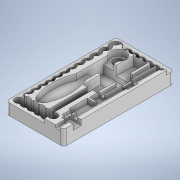
# Autodesk Inventor part: tool box
Saved by Autodesk Inventor 2020 (Build 240168000, 168)
## iProperties
Created: 2020-01-06
Part Number: tool box
Material: Générique
Document SubType Name: Modeling
Designer: damien
Density: 1 g/cm^3
Appearance: Par défaut
Author: damien
Autodesk Inventor part; units mm, degrees
ref_plane "YZ Plane" through (0, 0, 0) normal (1, 0, 0) x (0, 1, 0)
ref_plane "XZ Plane" through (0, 0, 0) normal (0, 1, 0) x (-1, 0, 0)
ref_plane "XY Plane" through (0, 0, 0) normal (0, 0, 1) x (1, 0, 0)
sketch "Esquisse1" plane through (0, 0, 0) normal (0, 1, 0) x (-1, 0, 0)
  line L0 (-50, -95.5) -> (50, -95.5)
  line L1 (50, -95.5) -> (50, 95.5)
  line L2 (50, 95.5) -> (-50, 95.5)
  line L3 (-50, 95.5) -> (-50, -95.5)
  line L4 (-50, -95.5) -> (50, 95.5) construction
  line L5 (50, -95.5) -> (-50, 95.5) construction
  point P0 (0, 0)
  dimension "d0" = 100
  dimension "d1" = 191
  constraints: 12 end point, 2 midpoint, 2 parallel, 1 horizontal, 1 perpendicular
  measures "d0" distance of L0.start L0.end
  measures "d1" distance of L0.end L1.end
extrude "Extrusion1" add sketch "Esquisse1" along normal blind 26.5
fillet "Congé1" radius 5 4 edges at (50, 13.25, 95.5) (50, 13.25, -95.5) (-50, 13.25, -95.5) (-50, 13.25, 95.5)
sketch "Esquisse2" plane through (0, 26.5, 0) normal (0, 1, 0) x (1, 0, 0)
  line L0 (-50, -95.5) -> (16.5, -95.5)
  line L1 (50, 95.5) -> (-50, 95.5)
  line L2 (-50, 95.5) -> (-50, -95.5)
  line L3 (50, 95.5) -> (-50, 95.5) projected
  line L4 (-50, 95.5) -> (-50, -95.5) projected
  line L5 (-50, -95.5) -> (50, -95.5) projected
  line L6 (-37, -80) -> (16.5, -80)
  line L7 (50, 82.5) -> (-37, 82.5)
  line L8 (-37, 82.5) -> (-37, -80)
  line L9 (16.5, -95.5) -> (16.5, -80)
  line L10 (50, 82.5) -> (50, 95.5)
  line L11 (50, -95.5) -> (50, 95.5) projected
  point P0 (0, 0)
  point P1 (45, 95.5)
  point P2 (-45, 95.5)
  point P3 (-50, 90.5)
  point P4 (45, -95.5)
  point P5 (50, -90.5)
  point P6 (50, 90.5)
  dimension "d5" = 15.5
  dimension "d7" = 13
  dimension "d8" = 13
  dimension "d9" = 66.5
  constraints: 19 end point, 4 parallel, 2 horizontal, 2 perpendicular, 1 collinear
  measures "d5" distance between parallel lines of L0 L6
  measures "d7" distance between parallel lines of L2 L8
  measures "d8" distance from line of point (45, 95.5) L7
  measures "d9" distance of L0.start L0.end
extrude "Extrusion2" cut sketch "Esquisse2" against normal blind 7 contours L2 L1 L10 L7 L8 L6 L9 L0
sketch "Esquisse4" plane through (0, 26.5, 0) normal (0, 1, 0) x (1, 0, 0)
  arc A0 (14, -87.1056) -> (14, -79.8944) centre (20, -83.5) ccw
  line L0 (50, -95.5) -> (50, 82.5) projected
  line L1 (16.5, -95.5) -> (50, -95.5) projected
  arc A1 (-34, -79.8944) -> (-34, -87.1056) centre (-40, -83.5) ccw
  line L2 (8, -83.5) -> (-4, -83.5) construction
  line L3 (-4, -83.5) -> (-16, -83.5) construction
  line L4 (-16, -83.5) -> (-28, -83.5) construction
  line L5 (-28, -83.5) -> (-40, -83.5) construction
  line L6 (-50, -90.5) -> (-50, 90.5) projected
  arc A2 (-34, -87.1056) -> (-22, -87.1056) centre (-28, -83.5) ccw
  arc A3 (-22, -79.8944) -> (-34, -79.8944) centre (-28, -83.5) ccw
  arc A4 (-22, -87.1056) -> (-10, -87.1056) centre (-16, -83.5) ccw
  arc A5 (-10, -79.8944) -> (-22, -79.8944) centre (-16, -83.5) ccw
  arc A6 (-10, -87.1056) -> (2, -87.1056) centre (-4, -83.5) ccw
  arc A7 (2, -79.8944) -> (-10, -79.8944) centre (-4, -83.5) ccw
  arc A8 (2, -87.1056) -> (14, -87.1056) centre (8, -83.5) ccw
  arc A9 (14, -79.8944) -> (2, -79.8944) centre (8, -83.5) ccw
  point P0 (0, 0)
  point P1 (50, -90.5)
  point P2 (45, -95.5)
  point P3 (-50, -95.5)
  point P4 (-50, 95.5)
  dimension "d12" = 30
  dimension "d13" = 14
  dimension "d14" = 12
  dimension "d16" = 12
  dimension "d17" = 12
  dimension "d18" = 12
  dimension "d19" = 12
  dimension "d20" = 12
  dimension "d21" = 10
  dimension "d25" = 14
  dimension "d26" = 7
  dimension "d27" = 7
  dimension "d28" = 7
  dimension "d29" = 7
  dimension "d30" = 7
  dimension "d31" = 7
  dimension "d32" = 7
  dimension "d33" = 7
  constraints: 20 point on circle, 10 centre point, 8 end point, 4 horizontal alignment, 3 collinear, 1 horizontal
  measures "d12" distance from line of L0 A0.centre
  measures "d13" diameter of A0
  measures "d14" distance from line of L1 A0.centre
  measures "d16" distance of A0.centre L2.start
  measures "d17" distance of L2.end L2.start
  measures "d18" distance of L2.end L3.end
  measures "d19" distance of L3.end L4.end
  measures "d20" distance of L4.end L5.end
  measures "d21" distance from line of L6 L5.end
  measures "d25" diameter of A1
  measures "d26" radius of A3
  measures "d27" radius of A2
  measures "d28" radius of A4
  measures "d29" radius of A5
  measures "d30" radius of A6
  measures "d31" radius of A7
  measures "d32" radius of A8
  measures "d33" radius of A9
extrude "Extrusion3" cut sketch "Esquisse4" against normal blind 26
fillet "Congé2" radius 2 10 edges at (-34, 13.5, 79.8944) (-22, 13.5, 79.8944) (-10, 13.5, 79.8944) (2, 13.5, 79.8944) (14, 13.5, 79.8944) (14, 10, 87.1056) (2, 10, 87.1056) (-10, 10, 87.1056) (-22, 10, 87.1056) (-34, 10, 87.1056)
fillet "Congé3" [suppressed]
sketch "Esquisse5" plane through (0, 26.5, 0) normal (0, 1, 0) x (1, 0, 0)
  arc A0 (-40.2854, -61.75) -> (-36.7146, -61.75) centre (-38.5, -68) ccw
  arc A1 (-36.619, 74.0454) -> (-40.381, 74.0454) centre (-38.5, 83) ccw
  arc A2 (-37, -77.1754) -> (-34, -87.1056) centre (-40, -83.5) ccw projected
  line L0 (-50, -90.5) -> (-50, 90.5) projected
  arc A3 (-36.7146, -61.75) -> (-36.7146, -49.25) centre (-38.5, -55.5) ccw
  arc A4 (-40.2854, -49.25) -> (-40.2854, -61.75) centre (-38.5, -55.5) ccw
  arc A5 (-36.7146, -49.25) -> (-36.7146, -36.75) centre (-38.5, -43) ccw
  arc A6 (-40.2854, -36.75) -> (-40.2854, -49.25) centre (-38.5, -43) ccw
  arc A7 (-36.7146, -36.75) -> (-36.7146, -24.25) centre (-38.5, -30.5) ccw
  arc A8 (-40.2854, -24.25) -> (-40.2854, -36.75) centre (-38.5, -30.5) ccw
  arc A9 (-36.7146, -24.25) -> (-36.7146, -11.75) centre (-38.5, -18) ccw
  arc A10 (-40.2854, -11.75) -> (-40.2854, -24.25) centre (-38.5, -18) ccw
  arc A11 (-36.7146, -11.75) -> (-36.7146, 0.75) centre (-38.5, -5.5) ccw
  arc A12 (-40.2854, 0.75) -> (-40.2854, -11.75) centre (-38.5, -5.5) ccw
  arc A13 (-36.7146, 0.75) -> (-36.9688, 13.3171) centre (-38.5, 7) ccw
  arc A14 (-40.0312, 13.3171) -> (-40.2854, 0.75) centre (-38.5, 7) ccw
  arc A15 (-36.9688, 13.3171) -> (-36.613, 27.0946) centre (-38.5, 20.25) ccw
  arc A16 (-40.387, 27.0946) -> (-40.0312, 13.3171) centre (-38.5, 20.25) ccw
  arc A17 (-36.613, 27.0946) -> (-36.5496, 41.3883) centre (-38.5, 34.25) ccw
  arc A18 (-40.4504, 41.3883) -> (-40.387, 27.0946) centre (-38.5, 34.25) ccw
  arc A19 (-36.5496, 41.3883) -> (-36.2736, 57.038) centre (-38.5, 49.25) ccw
  arc A20 (-40.7264, 57.038) -> (-40.4504, 41.3883) centre (-38.5, 49.25) ccw
  arc A21 (-36.2736, 57.038) -> (-36.619, 74.0454) centre (-38.5, 65.5) ccw
  arc A22 (-40.381, 74.0454) -> (-40.7264, 57.038) centre (-38.5, 65.5) ccw
  point P0 (0, 0)
  point P1 (-35.3333, -88.7175)
  point P2 (-35.3333, -78.2825)
  point P3 (-50, -95.5)
  point P4 (-50, 95.5)
  dimension "d38" = 13
  dimension "d39" = 15.5
  dimension "d40" = 7
  dimension "d41" = 11.5
  dimension "d42" = 12.5
  dimension "d43" = 12.5
  dimension "d44" = 12.5
  dimension "d45" = 12.5
  dimension "d46" = 12.5
  dimension "d47" = 6.5
  dimension "d49" = 12.5
  dimension "d51" = 13.25
  dimension "d52" = 14
  dimension "d55" = 15
  dimension "d57" = 16.25
  dimension "d58" = 18.3
  dimension "d59" = 17.5
  dimension "d60" = 6.5
  dimension "d61" = 6.5
  dimension "d62" = 7.1
  dimension "d63" = 7.4
  dimension "d64" = 8.1
  dimension "d65" = 8.75
  constraints: 44 point on circle, 22 centre point, 13 equal radius, 11 vertical alignment
  measures "d38" diameter of A0
  measures "d39" vertical distance of A2.centre A0.centre
  measures "d40" radius of A2
  measures "d41" distance from line of L0 A0.centre
  measures "d42" distance of A3.centre A0.centre
  measures "d43" distance of A5.centre A3.centre
  measures "d44" distance of A7.centre A5.centre
  measures "d45" distance of A9.centre A7.centre
  measures "d46" distance of A11.centre A9.centre
  measures "d47" radius of A3
  measures "d49" distance of A13.centre A11.centre
  measures "d51" distance of A13.centre A15.centre
  measures "d52" distance of A15.centre A17.centre
  measures "d55" distance of A17.centre A19.centre
  measures "d57" distance of A19.centre A21.centre
  measures "d58" diameter of A1
  measures "d59" distance of A21.centre A1.centre
  measures "d60" radius of A12
  measures "d61" radius of A14
  measures "d62" radius of A16
  measures "d63" radius of A18
  measures "d64" radius of A20
  measures "d65" radius of A22
extrude "Extrusion4" cut sketch "Esquisse5" against normal blind 26
fillet "Congé4" radius 2 10 edges at (-36.7146, 13.5, 49.25) (-36.7146, 13.5, 36.75) (-36.7146, 13.5, 24.25) (-36.7146, 13.5, 11.75) (-36.7146, 13.5, -0.75) (-36.9688, 13.5, -13.3171) (-36.613, 13.5, -27.0946) (-36.5496, 13.5, -41.3883) (-36.2736, 13.5, -57.038) (-36.619, 13.5, -74.0454)
fillet "Congé5" radius 2 12 edges at (-36.7146, 13.5, 61.75) (-40.2854, 10, 61.75) (-40.2854, 10, 49.25) (-40.2854, 10, 36.75) (-40.2854, 10, 24.25) (-40.2854, 10, 11.75) (-40.2854, 10, -0.75) (-40.0312, 10, -13.3171) (-40.387, 10, -27.0946) (-40.4504, 10, -41.3883) (-40.7264, 10, -57.038) (-40.381, 10, -74.0454)
fillet "Congé6" [suppressed]
sketch "Esquisse6" plane through (0, 26.5, 0) normal (0, 1, 0) x (1, 0, 0)
  arc A0 (-13, 85) -> (-13, 81.5) centre (-19, 83.25) ccw
  arc A1 (35, 81.5) -> (35, 85) centre (41, 83.25) ccw
  line L0 (-45, 95.5) -> (45, 95.5) projected
  line L1 (50, 90.5) -> (50, 82.5) projected
  arc A2 (-13, 81.5) -> (-1, 81.5) centre (-7, 83.25) ccw
  arc A3 (-1, 85) -> (-13, 85) centre (-7, 83.25) ccw
  arc A4 (-1, 81.5) -> (11, 81.5) centre (5, 83.25) ccw
  arc A5 (11, 85) -> (-1, 85) centre (5, 83.25) ccw
  arc A6 (11, 81.5) -> (23, 81.5) centre (17, 83.25) ccw
  arc A7 (23, 85) -> (11, 85) centre (17, 83.25) ccw
  arc A8 (23, 81.5) -> (35, 81.5) centre (29, 83.25) ccw
  arc A9 (35, 85) -> (23, 85) centre (29, 83.25) ccw
  point P0 (0, 0)
  point P1 (-50, 95.5)
  point P2 (50, 95.5)
  dimension "d71" = 12.5
  dimension "d72" = 12.25
  dimension "d73" = 12
  dimension "d74" = 12
  dimension "d75" = 12
  dimension "d76" = 12
  dimension "d77" = 12
  dimension "d78" = 9
  dimension "d79" = 6.25
  constraints: 20 point on circle, 10 centre point, 8 equal radius, 5 horizontal alignment
  measures "d71" diameter of A0
  measures "d72" distance from line of L0 A0.centre
  measures "d73" distance of A2.centre A0.centre
  measures "d74" distance of A4.centre A2.centre
  measures "d75" distance of A4.centre A6.centre
  measures "d76" distance of A6.centre A8.centre
  measures "d77" distance of A8.centre A1.centre
  measures "d78" distance from line of L1 A1.centre
  measures "d79" radius of A2
extrude "Extrusion5" cut sketch "Esquisse6" against normal blind 26
fillet "Congé7" radius 2 10 edges at (-13, 13.5, -81.5) (-1, 13.5, -81.5) (11, 13.5, -81.5) (23, 13.5, -81.5) (35, 13.5, -81.5) (35, 10, -85) (23, 10, -85) (11, 10, -85) (-1, 10, -85) (-13, 10, -85)
fillet "Congé8" [suppressed]
fillet "Congé9" [suppressed]
sketch "Esquisse7" plane through (0, 26.5, 0) normal (0, 1, 0) x (1, 0, 0)
  arc A0 (-5.5, 54.3692) -> (-23.5, 54.3692) centre (-14.5, 63.75) ccw
  line L0 (-23.5, 54.3692) -> (-23.5, -0.6308)
  arc A1 (-23.5, -0.6308) -> (-23.5, -69.9643) centre (60.5, -35.2976) ccw
  arc A2 (-5.5, -69.9643) -> (-5.5, -0.6308) centre (-89.5, -35.2976) ccw
  line L1 (-5.5, -0.6308) -> (-5.5, 54.3692)
  arc A3 (-23.5, -69.9643) -> (-5.5, -69.9643) centre (-14.5, -66.25) ccw
  line L2 (-14.5, -66.25) -> (-14.5, 63.75) construction
  arc A4 (-40.2854, -61.75) -> (-37, -74.3246) centre (-38.5, -68) ccw projected
  arc A5 (-25.2048, 82.5) -> (-13, 81.5) centre (-19, 83.25) ccw projected
  point P0 (0, 0)
  dimension "d85" = 18
  dimension "d88" = 26
  dimension "d89" = 130
  dimension "d102" = 90.8723
  dimension "d103" = 150
  dimension "d104" = 55
  dimension "d156" = 24
  dimension "d157" = 19.5
  constraints: 8 point on circle, 6 end point, 4 centre point, 3 vertical, 2 tangent, 1 equal radius, 1 horizontal alignment, 1 parallel, 1 vertical alignment
  measures "d85" distance between parallel lines of L1 L0
  measures "d88" diameter of A0
  measures "d89" distance of L2.end L2.start
  measures "d102" radius of A1
  measures "d103" distance of A1.centre A2.centre
  measures "d104" distance of L1.start L1.end
  measures "d156" distance from line of L2 A4.centre
  measures "d157" vertical distance of A5.centre L2.end
extrude "Extrusion6" cut sketch "Esquisse7" against normal blind 10.5
sketch "Esquisse8" plane through (0, 16, 0) normal (0, 1, 0) x (1, 0, 0)
  arc A0 (-5.5, 54.3692) -> (-23.5, 54.3692) centre (-14.5, 63.75) ccw projected
  circle A1 centre (-14.5, 63.75) radius 8.5
  point P0 (0, 0)
  point P1 (-8.1285, 76.0884)
  dimension "d97" = 17
  constraints: 1 centre point, 1 coincident
  measures "d97" diameter of A1
extrude "Extrusion7" cut sketch "Esquisse8" against normal blind 15
sketch "Esquisse9" plane through (0, 26.5, 0) normal (0, 1, 0) x (1, 0, 0)
  line L0 (-1, 76.75) -> (23, 76.75)
  line L1 (23, 76.75) -> (23, -11.25)
  line L2 (-1, -11.25) -> (-1, 76.75)
  line L3 (6.5, -11.25) -> (6.5, -80.25)
  line L4 (6.5, -80.25) -> (15.5, -80.25)
  line L5 (15.5, -80.25) -> (15.5, -11.25)
  line L6 (15.5, -11.25) -> (23, -11.25)
  line L7 (-1, -11.25) -> (6.5, -11.25)
  line L8 (-5.5, 54.3692) -> (-5.5, -0.6308) projected
  arc A0 (-1, 81.5) -> (11, 81.5) centre (5, 83.25) ccw projected
  dimension "d106" = 9
  dimension "d109" = 69
  dimension "d110" = 88
  dimension "d111" = 24
  dimension "d113" = 4.5
  dimension "d158" = 6.5
  constraints: 16 end point, 4 parallel, 3 horizontal, 3 perpendicular, 2 collinear
  measures "d106" distance of L3.end L4.end
  measures "d109" distance of L4.end L5.end
  measures "d110" distance of L0.end L1.end
  measures "d111" distance of L0.start L0.end
  measures "d113" distance between parallel lines of L8 L2
  measures "d158" distance from line of A0.centre L0
extrude "Extrusion8" cut sketch "Esquisse9" against normal blind 16
sketch "Esquisse10" plane through (0, 26.5, 0) normal (0, 1, 0) x (1, 0, 0)
  line L0 (-23.5, -0.6308) -> (-23.5, 54.3692) projected
  line L1 (-23.5, 19) -> (30.5, 19)
  line L2 (30.5, 19) -> (30.5, 47)
  line L3 (30.5, 47) -> (-23.5, 47)
  line L4 (-23.5, 47) -> (-23.5, 19)
  line L5 (-45, 95.5) -> (45, 95.5) projected
  line L6 (50, -95.5) -> (50, 82.5) projected
  point P0 (0, 0)
  point P1 (50, -90.5)
  point P2 (-50, 95.5)
  point P3 (50, 95.5)
  dimension "d116" = 28
  dimension "d117" = 48.5
  dimension "d118" = 19.5
  constraints: 8 end point, 2 parallel, 1 horizontal, 1 perpendicular, 1 point on line
  measures "d116" distance of L1.end L2.end
  measures "d117" distance between parallel lines of L5 L3
  measures "d118" distance between parallel lines of L6 L2
extrude "Extrusion9" cut sketch "Esquisse10" against normal blind 25
sketch "Esquisse11" plane through (0, 26.5, 0) normal (0, 1, 0) x (1, 0, 0)
  line L0 (-50, -95.5) -> (50, -95.5) projected
  line L1 (43, -95.5) -> (36, -95.5)
  line L2 (36, -95.5) -> (36, 82)
  line L3 (36, 82) -> (43, 82)
  line L4 (43, 82) -> (43, -95.5)
  line L5 (50, -95.5) -> (50, 82.5) projected
  line L6 (34, 82) -> (27, 82)
  line L7 (27, 82) -> (27, -8.75)
  line L8 (27, -8.75) -> (34, -8.75)
  line L9 (34, -8.75) -> (34, 82)
  line L10 (23, 76.75) -> (23, 47) projected
  arc A0 (23, 81.5) -> (35, 81.5) centre (29, 83.25) ccw projected
  point P0 (0, 0)
  point P1 (-45, -95.5)
  point P2 (45, -95.5)
  point P3 (50, -90.5)
  dimension "d122" = 7
  dimension "d123" = 7
  dimension "d126" = 92
  dimension "d128" = 4
  dimension "d129" = 7
  dimension "d159" = 1.25
  constraints: 16 end point, 4 parallel, 2 horizontal, 2 perpendicular, 1 collinear, 1 point on line
  measures "d122" distance of L2.end L3.end
  measures "d123" distance between parallel lines of L5 L4
  measures "d126" distance from line of point (29, 83.25) L8
  measures "d128" distance between parallel lines of L10 L7
  measures "d129" distance between parallel lines of L9 L7
  measures "d159" distance from line of A0.centre L6
extrude "Extrusion10" cut sketch "Esquisse11" against normal blind 5
sketch "Esquisse12" plane through (0, 26.5, 0) normal (0, 1, 0) x (1, 0, 0)
  line L0 (36, -95.5) -> (36, 79.3197) projected
  line L1 (24, -8.75) -> (36, -8.75)
  line L2 (36, -8.75) -> (36, -24.75)
  line L3 (36, -24.75) -> (24, -24.75)
  line L4 (24, -24.75) -> (24, -8.75)
  line L5 (34, -8.75) -> (27, -8.75) projected
  line L6 (36, -27.75) -> (23, -27.75)
  line L7 (23, -27.75) -> (23, -59.75)
  line L8 (23, -59.75) -> (36, -59.75)
  line L9 (36, -59.75) -> (36, -27.75)
  line L10 (45.5, 38.25) -> (33.5, 38.25)
  line L11 (33.5, 38.25) -> (33.5, 20.25)
  line L12 (33.5, 20.25) -> (45.5, 20.25)
  line L13 (45.5, 20.25) -> (45.5, 38.25)
  arc A0 (36.4545, 78.9603) -> (43, 77.3286) centre (41, 83.25) ccw projected
  line L14 (43, 77.3286) -> (43, -95.5) projected
  line L15 (27, -8.75) -> (27, 19) projected
  line L16 (50, -95.5) -> (50, 82.5) projected
  line L17 (50, -79.5) -> (30, -79.5)
  line L18 (30, -79.5) -> (30, -65.5)
  line L19 (30, -65.5) -> (50, -65.5)
  line L20 (50, -65.5) -> (50, -79.5)
  line L21 (43, -95.5) -> (36, -95.5) projected
  point P0 (0, 0)
  point P1 (36, 78.7057)
  point P2 (43, 76.8031)
  point P3 (50, -90.5)
  point P4 (36, 79.5)
  dimension "d132" = 16
  dimension "d133" = 12
  dimension "d134" = 32
  dimension "d135" = 3
  dimension "d136" = 13
  dimension "d137" = 45
  dimension "d138" = 18
  dimension "d139" = 12
  dimension "d140" = 2.5
  dimension "d141" = 2.5
  dimension "d142" = 3
  dimension "d143" = 16
  dimension "d144" = 14
  dimension "d145" = 20
  constraints: 32 end point, 8 parallel, 4 horizontal, 4 perpendicular, 3 point on line, 1 collinear
  measures "d132" distance of L3.end L1.start
  measures "d133" distance of L2.end L3.end
  measures "d134" distance of L6.end L7.end
  measures "d135" distance between parallel lines of L3 L6
  measures "d136" distance of L7.end L8.end
  measures "d137" distance from line of A0.centre L10
  measures "d138" distance of L12.end L10.start
  measures "d139" distance of L10.start L10.end
  measures "d140" distance between parallel lines of L14 L13
  measures "d141" distance between parallel lines of L0 L11
  measures "d142" distance between parallel lines of L15 L4
  measures "d143" distance between parallel lines of L21 L17
  measures "d144" distance of L19.end L17.start
  measures "d145" distance of L18.end L19.end
extrude "Extrusion11" cut sketch "Esquisse12" against normal blind 9 contours L8 L7 L6 L0 | L19 L14 L17 L0 | L0 L17 L18 L19 | L3 L4 L1 L0 | L19 L16 L17 L14 | L14 L10 L13 L12 | L12 L0 L10 L14 | L12 L11 L10 L0
sketch "Esquisse13" plane through (0, 26.5, 0) normal (0, 1, 0) x (1, 0, 0)
  line L0 (36, -59.75) -> (23, -59.75) projected
  line L1 (33, -59.75) -> (26, -59.75)
  line L2 (26, -59.75) -> (26, -74.75)
  line L3 (26, -74.75) -> (33, -74.75)
  line L4 (33, -74.75) -> (33, -59.75)
  line L5 (23, -59.75) -> (23, -27.75) projected
  line L6 (36, -59.75) -> (36, -27.75) projected
  point P0 (0, 0)
  dimension "d148" = 3
  dimension "d149" = 7
  dimension "d150" = 15
  dimension "d151" = 3
  constraints: 8 end point, 2 parallel, 1 horizontal, 1 perpendicular, 1 point on line
  measures "d148" distance between parallel lines of L5 L2
  measures "d149" distance of L2.end L3.end
  measures "d150" distance of L3.end L1.start
  measures "d151" distance between parallel lines of L4 L6
extrude "Extrusion12" cut sketch "Esquisse13" against normal blind 5
fillet "Congé12" [suppressed]
fillet "Congé13" [suppressed]
